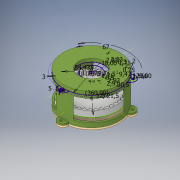
# Autodesk Inventor part: HarmonicDriveProto2
Saved by Autodesk Inventor 2018.3 (Build 223284000, 284)
## iProperties
Created: 2018-06-22
Part Number: HarmonicDriveProto2
Material: Generisch
Document SubType Name: Modeling
Designer: JochenAlt
Density: 1 g/cm^3
Appearance: Vorgabe
Author: JochenAlt
Autodesk Inventor part; units mm, degrees
note: some values were not read from the file. Chosen so that the rebuilt part matches the saved one: sketch regions of "Extrusion4".
(part 1 of 2)
sketch "Riemen" plane through (0, 0, 0) normal (0, 0, 1) x (1, 0, 0)
  circle A0 centre (0, 0) radius 26.0231 construction
  circle A1 centre (0, 0) radius 25.0331
  circle A2 centre (0, 0) radius 27.7331 construction
  line L0 (0, 43.2011) -> (0, -39.5773) construction
  line L1 (-38.8525, 0) -> (38.8525, 0) construction
  line L2 (0, 0) -> (5.5324, 31.3756) construction
  circle A3 centre (0, 0) radius 25.7831 construction
  line L3 (-1.465, 25.7414) -> (1.465, 25.7414) construction
  line L4 (3.0272, 25.6048) -> (5.9127, 25.096) construction
  arc A4 (4.0244, 27.3363) -> (3.1484, 26.0672) centre (5.9127, 25.096) ccw
  arc A5 (0.5595, 27.7275) -> (0, 27.7331) centre (0, 0) ccw
  arc A6 (4.8158, 27.3118) -> (4.2638, 27.4034) centre (0, 0) ccw
  arc A7 (2.8327, 25.8685) -> (1.7024, 25.9674) centre (0, 0) ccw
  arc A8 (1.426, 26.2179) -> (0.7837, 27.6198) centre (-1.465, 25.7414) ccw
  arc A9 (0.7837, 27.6198) -> (0.5595, 27.7275) centre (0.5534, 27.4275) ccw
  arc A10 (1.426, 26.2179) -> (1.7024, 25.9674) centre (1.722, 26.2667) ccw
  arc A11 (2.8327, 25.8685) -> (3.1484, 26.0672) centre (2.8653, 26.1667) ccw
  arc A12 (4.2638, 27.4034) -> (4.0244, 27.3363) centre (4.2177, 27.1069) ccw
  line L5 (0, 0) -> (2.7172, 31.0575) construction
  arc A13 (-4.2638, 27.4034) -> (-4.8158, 27.3118) centre (0, 0) ccw
  arc A14 (-4.0244, 27.3363) -> (-4.2638, 27.4034) centre (-4.2177, 27.1069) ccw
  arc A15 (-3.1484, 26.0672) -> (-4.0244, 27.3363) centre (-5.9127, 25.096) ccw
  arc A16 (-3.1484, 26.0672) -> (-2.8327, 25.8685) centre (-2.8653, 26.1667) ccw
  arc A17 (-1.7024, 25.9674) -> (-2.8327, 25.8685) centre (0, 0) ccw
  arc A18 (-1.7024, 25.9674) -> (-1.426, 26.2179) centre (-1.722, 26.2667) ccw
  arc A19 (-0.7837, 27.6198) -> (-1.426, 26.2179) centre (1.465, 25.7414) ccw
  arc A20 (-0.5595, 27.7275) -> (-0.7837, 27.6198) centre (-0.5534, 27.4275) ccw
  arc A21 (0, 27.7331) -> (-0.5595, 27.7275) centre (0, 0) ccw
  arc A22 (-8.9576, 26.2466) -> (-9.4853, 26.0606) centre (0, 0) ccw
  arc A23 (-8.7101, 26.2222) -> (-8.9576, 26.2466) centre (-8.8607, 25.9627) ccw
  arc A24 (-7.6271, 25.1245) -> (-8.7101, 26.2222) centre (-10.1807, 23.688) ccw
  arc A25 (-7.6271, 25.1245) -> (-7.2816, 24.9836) centre (-7.3656, 25.2716) ccw
  arc A26 (-6.1857, 25.2772) -> (-7.2816, 24.9836) centre (0, 0) ccw
  arc A27 (-6.1857, 25.2772) -> (-5.957, 25.572) centre (-6.257, 25.5686) ccw
  arc A28 (-5.5679, 27.0642) -> (-5.957, 25.572) centre (-3.0272, 25.6048) ccw
  arc A29 (-5.3658, 27.2091) -> (-5.5679, 27.0642) centre (-5.3078, 26.9147) ccw
  arc A30 (-4.8158, 27.3118) -> (-5.3658, 27.2091) centre (0, 0) ccw
  arc A31 (-13.3792, 24.2924) -> (-13.8666, 24.0176) centre (0, 0) ccw
  arc A32 (-13.1312, 24.3113) -> (-13.3792, 24.2924) centre (-13.2345, 24.0296) ccw
  arc A33 (-11.874, 23.4184) -> (-13.1312, 24.3113) centre (-14.1395, 21.5602) ccw
  arc A34 (-11.874, 23.4184) -> (-11.5094, 23.3396) centre (-11.6421, 23.6086) ccw
  arc A35 (-10.4811, 23.8191) -> (-11.5094, 23.3396) centre (0, 0) ccw
  arc A36 (-10.4811, 23.8191) -> (-10.3071, 24.1491) centre (-10.6019, 24.0937) ccw
  arc A37 (-10.183, 25.6861) -> (-10.3071, 24.1491) centre (-7.4274, 24.6901) ccw
  arc A38 (-10.0091, 25.8639) -> (-10.183, 25.6861) centre (-9.9008, 25.5842) ccw
  arc A39 (-9.4853, 26.0606) -> (-10.0091, 25.8639) centre (0, 0) ccw
  arc A40 (-17.3943, 21.6001) -> (-17.8265, 21.2448) centre (0, 0) ccw
  arc A41 (-17.1534, 21.6618) -> (-17.3943, 21.6001) centre (-17.2061, 21.3664) ccw
  arc A42 (-15.7602, 21.0007) -> (-17.1534, 21.6618) centre (-17.6685, 18.7774) ccw
  arc A43 (-15.7602, 21.0007) -> (-15.3874, 20.9864) centre (-15.5648, 21.2284) ccw
  arc A44 (-14.458, 21.6372) -> (-15.3874, 20.9864) centre (0, 0) ccw
  arc A45 (-14.458, 21.6372) -> (-14.3439, 21.9924) centre (-14.6247, 21.8866) ccw
  arc A46 (-14.4886, 23.5277) -> (-14.3439, 21.9924) centre (-11.602, 23.0252) ccw
  arc A47 (-14.3483, 23.7329) -> (-14.4886, 23.5277) centre (-14.193, 23.4762) ccw
  arc A48 (-13.8666, 24.0176) -> (-14.3483, 23.7329) centre (0, 0) ccw
  arc A49 (-20.8808, 18.2515) -> (-21.2448, 17.8265) centre (0, 0) ccw
  arc A50 (-20.6543, 18.354) -> (-20.8808, 18.2515) centre (-20.655, 18.054) ccw
  arc A51 (-19.1675, 17.9449) -> (-20.6543, 18.354) centre (-20.6608, 15.424) ccw
  arc A52 (-19.1675, 17.9449) -> (-18.7979, 17.9956) centre (-19.0146, 18.2031) ccw
  arc A53 (-17.9956, 18.7979) -> (-18.7979, 17.9956) centre (0, 0) ccw
  arc A54 (-17.9956, 18.7979) -> (-17.9449, 19.1675) centre (-18.2031, 19.0146) ccw
  arc A55 (-18.354, 20.6543) -> (-17.9449, 19.1675) centre (-15.424, 20.6608) ccw
  arc A56 (-18.2515, 20.8808) -> (-18.354, 20.6543) centre (-18.054, 20.655) ccw
  arc A57 (-17.8265, 21.2448) -> (-18.2515, 20.8808) centre (0, 0) ccw
  arc A58 (-23.7329, 14.3483) -> (-24.0176, 13.8666) centre (0, 0) ccw
  arc A59 (-23.5277, 14.4886) -> (-23.7329, 14.3483) centre (-23.4762, 14.193) ccw
  arc A60 (-21.9924, 14.3439) -> (-23.5277, 14.4886) centre (-23.0252, 11.602) ccw
  arc A61 (-21.9924, 14.3439) -> (-21.6372, 14.458) centre (-21.8866, 14.6247) ccw
  arc A62 (-20.9864, 15.3874) -> (-21.6372, 14.458) centre (0, 0) ccw
  arc A63 (-20.9864, 15.3874) -> (-21.0007, 15.7602) centre (-21.2284, 15.5648) ccw
  arc A64 (-21.6618, 17.1534) -> (-21.0007, 15.7602) centre (-18.7774, 17.6685) ccw
  arc A65 (-21.6001, 17.3943) -> (-21.6618, 17.1534) centre (-21.3664, 17.2061) ccw
  arc A66 (-21.2448, 17.8265) -> (-21.6001, 17.3943) centre (0, 0) ccw
  arc A67 (-25.8639, 10.0091) -> (-26.0606, 9.4853) centre (0, 0) ccw
  arc A68 (-25.6861, 10.183) -> (-25.8639, 10.0091) centre (-25.5842, 9.9008) ccw
  arc A69 (-24.1491, 10.3071) -> (-25.6861, 10.183) centre (-24.6901, 7.4274) ccw
  arc A70 (-24.1491, 10.3071) -> (-23.8191, 10.4811) centre (-24.0937, 10.6019) ccw
  arc A71 (-23.3396, 11.5094) -> (-23.8191, 10.4811) centre (0, 0) ccw
  arc A72 (-23.3396, 11.5094) -> (-23.4184, 11.874) centre (-23.6086, 11.6421) ccw
  arc A73 (-24.3113, 13.1312) -> (-23.4184, 11.874) centre (-21.5602, 14.1395) ccw
  arc A74 (-24.2924, 13.3792) -> (-24.3113, 13.1312) centre (-24.0296, 13.2345) ccw
  arc A75 (-24.0176, 13.8666) -> (-24.2924, 13.3792) centre (0, 0) ccw
  arc A76 (-27.2091, 5.3658) -> (-27.3118, 4.8158) centre (0, 0) ccw
  arc A77 (-27.0642, 5.5679) -> (-27.2091, 5.3658) centre (-26.9147, 5.3078) ccw
  arc A78 (-25.572, 5.957) -> (-27.0642, 5.5679) centre (-25.6048, 3.0272) ccw
  arc A79 (-25.572, 5.957) -> (-25.2772, 6.1857) centre (-25.5686, 6.257) ccw
  arc A80 (-24.9836, 7.2816) -> (-25.2772, 6.1857) centre (0, 0) ccw
  arc A81 (-24.9836, 7.2816) -> (-25.1245, 7.6271) centre (-25.2716, 7.3656) ccw
  arc A82 (-26.2222, 8.7101) -> (-25.1245, 7.6271) centre (-23.688, 10.1807) ccw
  arc A83 (-26.2466, 8.9576) -> (-26.2222, 8.7101) centre (-25.9627, 8.8607) ccw
  arc A84 (-26.0606, 9.4853) -> (-26.2466, 8.9576) centre (0, 0) ccw
  arc A85 (-27.7275, 0.5595) -> (-27.7331, 0) centre (0, 0) ccw
  arc A86 (-27.6198, 0.7837) -> (-27.7275, 0.5595) centre (-27.4275, 0.5534) ccw
  arc A87 (-26.2179, 1.426) -> (-27.6198, 0.7837) centre (-25.7414, -1.465) ccw
  arc A88 (-26.2179, 1.426) -> (-25.9674, 1.7024) centre (-26.2667, 1.722) ccw
  arc A89 (-25.8685, 2.8327) -> (-25.9674, 1.7024) centre (0, 0) ccw
  arc A90 (-25.8685, 2.8327) -> (-26.0672, 3.1484) centre (-26.1667, 2.8653) ccw
  arc A91 (-27.3363, 4.0244) -> (-26.0672, 3.1484) centre (-25.096, 5.9127) ccw
  arc A92 (-27.4034, 4.2638) -> (-27.3363, 4.0244) centre (-27.1069, 4.2177) ccw
  arc A93 (-27.3118, 4.8158) -> (-27.4034, 4.2638) centre (0, 0) ccw
  arc A94 (-27.4034, -4.2638) -> (-27.3118, -4.8158) centre (0, 0) ccw
  arc A95 (-27.3363, -4.0244) -> (-27.4034, -4.2638) centre (-27.1069, -4.2177) ccw
  arc A96 (-26.0672, -3.1484) -> (-27.3363, -4.0244) centre (-25.096, -5.9127) ccw
  arc A97 (-26.0672, -3.1484) -> (-25.8685, -2.8327) centre (-26.1667, -2.8653) ccw
  arc A98 (-25.9674, -1.7024) -> (-25.8685, -2.8327) centre (0, 0) ccw
  arc A99 (-25.9674, -1.7024) -> (-26.2179, -1.426) centre (-26.2667, -1.722) ccw
  arc A100 (-27.6198, -0.7837) -> (-26.2179, -1.426) centre (-25.7414, 1.465) ccw
  arc A101 (-27.7275, -0.5595) -> (-27.6198, -0.7837) centre (-27.4275, -0.5534) ccw
  arc A102 (-27.7331, 0) -> (-27.7275, -0.5595) centre (0, 0) ccw
  arc A103 (-26.2466, -8.9576) -> (-26.0606, -9.4853) centre (0, 0) ccw
  arc A104 (-26.2222, -8.7101) -> (-26.2466, -8.9576) centre (-25.9627, -8.8607) ccw
  arc A105 (-25.1245, -7.6271) -> (-26.2222, -8.7101) centre (-23.688, -10.1807) ccw
  arc A106 (-25.1245, -7.6271) -> (-24.9836, -7.2816) centre (-25.2716, -7.3656) ccw
  arc A107 (-25.2772, -6.1857) -> (-24.9836, -7.2816) centre (0, 0) ccw
  arc A108 (-25.2772, -6.1857) -> (-25.572, -5.957) centre (-25.5686, -6.257) ccw
  arc A109 (-27.0642, -5.5679) -> (-25.572, -5.957) centre (-25.6048, -3.0272) ccw
  arc A110 (-27.2091, -5.3658) -> (-27.0642, -5.5679) centre (-26.9147, -5.3078) ccw
  arc A111 (-27.3118, -4.8158) -> (-27.2091, -5.3658) centre (0, 0) ccw
  arc A112 (-24.2924, -13.3792) -> (-24.0176, -13.8666) centre (0, 0) ccw
  arc A113 (-24.3113, -13.1312) -> (-24.2924, -13.3792) centre (-24.0296, -13.2345) ccw
  arc A114 (-23.4184, -11.874) -> (-24.3113, -13.1312) centre (-21.5602, -14.1395) ccw
  arc A115 (-23.4184, -11.874) -> (-23.3396, -11.5094) centre (-23.6086, -11.6421) ccw
  arc A116 (-23.8191, -10.4811) -> (-23.3396, -11.5094) centre (0, 0) ccw
  arc A117 (-23.8191, -10.4811) -> (-24.1491, -10.3071) centre (-24.0937, -10.6019) ccw
  arc A118 (-25.6861, -10.183) -> (-24.1491, -10.3071) centre (-24.6901, -7.4274) ccw
  arc A119 (-25.8639, -10.0091) -> (-25.6861, -10.183) centre (-25.5842, -9.9008) ccw
  arc A120 (-26.0606, -9.4853) -> (-25.8639, -10.0091) centre (0, 0) ccw
  arc A121 (-21.6001, -17.3943) -> (-21.2448, -17.8265) centre (0, 0) ccw
  arc A122 (-21.6618, -17.1534) -> (-21.6001, -17.3943) centre (-21.3664, -17.2061) ccw
  arc A123 (-21.0007, -15.7602) -> (-21.6618, -17.1534) centre (-18.7774, -17.6685) ccw
  arc A124 (-21.0007, -15.7602) -> (-20.9864, -15.3874) centre (-21.2284, -15.5648) ccw
  arc A125 (-21.6372, -14.458) -> (-20.9864, -15.3874) centre (0, 0) ccw
  arc A126 (-21.6372, -14.458) -> (-21.9924, -14.3439) centre (-21.8866, -14.6247) ccw
  arc A127 (-23.5277, -14.4886) -> (-21.9924, -14.3439) centre (-23.0252, -11.602) ccw
  arc A128 (-23.7329, -14.3483) -> (-23.5277, -14.4886) centre (-23.4762, -14.193) ccw
  arc A129 (-24.0176, -13.8666) -> (-23.7329, -14.3483) centre (0, 0) ccw
  arc A130 (-18.2515, -20.8808) -> (-17.8265, -21.2448) centre (0, 0) ccw
  arc A131 (-18.354, -20.6543) -> (-18.2515, -20.8808) centre (-18.054, -20.655) ccw
  arc A132 (-17.9449, -19.1675) -> (-18.354, -20.6543) centre (-15.424, -20.6608) ccw
  arc A133 (-17.9449, -19.1675) -> (-17.9956, -18.7979) centre (-18.2031, -19.0146) ccw
  arc A134 (-18.7979, -17.9956) -> (-17.9956, -18.7979) centre (0, 0) ccw
  arc A135 (-18.7979, -17.9956) -> (-19.1675, -17.9449) centre (-19.0146, -18.2031) ccw
  arc A136 (-20.6543, -18.354) -> (-19.1675, -17.9449) centre (-20.6608, -15.424) ccw
  arc A137 (-20.8808, -18.2515) -> (-20.6543, -18.354) centre (-20.655, -18.054) ccw
  arc A138 (-21.2448, -17.8265) -> (-20.8808, -18.2515) centre (0, 0) ccw
  arc A139 (-14.3483, -23.7329) -> (-13.8666, -24.0176) centre (0, 0) ccw
  arc A140 (-14.4886, -23.5277) -> (-14.3483, -23.7329) centre (-14.193, -23.4762) ccw
  arc A141 (-14.3439, -21.9924) -> (-14.4886, -23.5277) centre (-11.602, -23.0252) ccw
  arc A142 (-14.3439, -21.9924) -> (-14.458, -21.6372) centre (-14.6247, -21.8866) ccw
  arc A143 (-15.3874, -20.9864) -> (-14.458, -21.6372) centre (0, 0) ccw
  arc A144 (-15.3874, -20.9864) -> (-15.7602, -21.0007) centre (-15.5648, -21.2284) ccw
  arc A145 (-17.1534, -21.6618) -> (-15.7602, -21.0007) centre (-17.6685, -18.7774) ccw
  arc A146 (-17.3943, -21.6001) -> (-17.1534, -21.6618) centre (-17.2061, -21.3664) ccw
  arc A147 (-17.8265, -21.2448) -> (-17.3943, -21.6001) centre (0, 0) ccw
  arc A148 (-10.0091, -25.8639) -> (-9.4853, -26.0606) centre (0, 0) ccw
  arc A149 (-10.183, -25.6861) -> (-10.0091, -25.8639) centre (-9.9008, -25.5842) ccw
  arc A150 (-10.3071, -24.1491) -> (-10.183, -25.6861) centre (-7.4274, -24.6901) ccw
  arc A151 (-10.3071, -24.1491) -> (-10.4811, -23.8191) centre (-10.6019, -24.0937) ccw
  arc A152 (-11.5094, -23.3396) -> (-10.4811, -23.8191) centre (0, 0) ccw
  arc A153 (-11.5094, -23.3396) -> (-11.874, -23.4184) centre (-11.6421, -23.6086) ccw
  arc A154 (-13.1312, -24.3113) -> (-11.874, -23.4184) centre (-14.1395, -21.5602) ccw
  arc A155 (-13.3792, -24.2924) -> (-13.1312, -24.3113) centre (-13.2345, -24.0296) ccw
  arc A156 (-13.8666, -24.0176) -> (-13.3792, -24.2924) centre (0, 0) ccw
  arc A157 (-5.3658, -27.2091) -> (-4.8158, -27.3118) centre (0, 0) ccw
  arc A158 (-5.5679, -27.0642) -> (-5.3658, -27.2091) centre (-5.3078, -26.9147) ccw
  arc A159 (-5.957, -25.572) -> (-5.5679, -27.0642) centre (-3.0272, -25.6048) ccw
  arc A160 (-5.957, -25.572) -> (-6.1857, -25.2772) centre (-6.257, -25.5686) ccw
  arc A161 (-7.2816, -24.9836) -> (-6.1857, -25.2772) centre (0, 0) ccw
  arc A162 (-7.2816, -24.9836) -> (-7.6271, -25.1245) centre (-7.3656, -25.2716) ccw
  arc A163 (-8.7101, -26.2222) -> (-7.6271, -25.1245) centre (-10.1807, -23.688) ccw
  arc A164 (-8.9576, -26.2466) -> (-8.7101, -26.2222) centre (-8.8607, -25.9627) ccw
  arc A165 (-9.4853, -26.0606) -> (-8.9576, -26.2466) centre (0, 0) ccw
  arc A166 (-0.5595, -27.7275) -> (0, -27.7331) centre (0, 0) ccw
  arc A167 (-0.7837, -27.6198) -> (-0.5595, -27.7275) centre (-0.5534, -27.4275) ccw
  arc A168 (-1.426, -26.2179) -> (-0.7837, -27.6198) centre (1.465, -25.7414) ccw
  arc A169 (-1.426, -26.2179) -> (-1.7024, -25.9674) centre (-1.722, -26.2667) ccw
  arc A170 (-2.8327, -25.8685) -> (-1.7024, -25.9674) centre (0, 0) ccw
  arc A171 (-2.8327, -25.8685) -> (-3.1484, -26.0672) centre (-2.8653, -26.1667) ccw
  arc A172 (-4.0244, -27.3363) -> (-3.1484, -26.0672) centre (-5.9127, -25.096) ccw
  arc A173 (-4.2638, -27.4034) -> (-4.0244, -27.3363) centre (-4.2177, -27.1069) ccw
  arc A174 (-4.8158, -27.3118) -> (-4.2638, -27.4034) centre (0, 0) ccw
  arc A175 (4.2638, -27.4034) -> (4.8158, -27.3118) centre (0, 0) ccw
  arc A176 (4.0244, -27.3363) -> (4.2638, -27.4034) centre (4.2177, -27.1069) ccw
  arc A177 (3.1484, -26.0672) -> (4.0244, -27.3363) centre (5.9127, -25.096) ccw
  arc A178 (3.1484, -26.0672) -> (2.8327, -25.8685) centre (2.8653, -26.1667) ccw
  arc A179 (1.7024, -25.9674) -> (2.8327, -25.8685) centre (0, 0) ccw
  arc A180 (1.7024, -25.9674) -> (1.426, -26.2179) centre (1.722, -26.2667) ccw
  arc A181 (0.7837, -27.6198) -> (1.426, -26.2179) centre (-1.465, -25.7414) ccw
  arc A182 (0.5595, -27.7275) -> (0.7837, -27.6198) centre (0.5534, -27.4275) ccw
  arc A183 (0, -27.7331) -> (0.5595, -27.7275) centre (0, 0) ccw
  arc A184 (8.9576, -26.2466) -> (9.4853, -26.0606) centre (0, 0) ccw
  arc A185 (8.7101, -26.2222) -> (8.9576, -26.2466) centre (8.8607, -25.9627) ccw
  arc A186 (7.6271, -25.1245) -> (8.7101, -26.2222) centre (10.1807, -23.688) ccw
  arc A187 (7.6271, -25.1245) -> (7.2816, -24.9836) centre (7.3656, -25.2716) ccw
  arc A188 (6.1857, -25.2772) -> (7.2816, -24.9836) centre (0, 0) ccw
  arc A189 (6.1857, -25.2772) -> (5.957, -25.572) centre (6.257, -25.5686) ccw
  arc A190 (5.5679, -27.0642) -> (5.957, -25.572) centre (3.0272, -25.6048) ccw
  arc A191 (5.3658, -27.2091) -> (5.5679, -27.0642) centre (5.3078, -26.9147) ccw
  arc A192 (4.8158, -27.3118) -> (5.3658, -27.2091) centre (0, 0) ccw
  arc A193 (13.3792, -24.2924) -> (13.8666, -24.0176) centre (0, 0) ccw
  arc A194 (13.1312, -24.3113) -> (13.3792, -24.2924) centre (13.2345, -24.0296) ccw
  arc A195 (11.874, -23.4184) -> (13.1312, -24.3113) centre (14.1395, -21.5602) ccw
  arc A196 (11.874, -23.4184) -> (11.5094, -23.3396) centre (11.6421, -23.6086) ccw
  arc A197 (10.4811, -23.8191) -> (11.5094, -23.3396) centre (0, 0) ccw
  arc A198 (10.4811, -23.8191) -> (10.3071, -24.1491) centre (10.6019, -24.0937) ccw
  arc A199 (10.183, -25.6861) -> (10.3071, -24.1491) centre (7.4274, -24.6901) ccw
  arc A200 (10.0091, -25.8639) -> (10.183, -25.6861) centre (9.9008, -25.5842) ccw
  arc A201 (9.4853, -26.0606) -> (10.0091, -25.8639) centre (0, 0) ccw
  arc A202 (17.3943, -21.6001) -> (17.8265, -21.2448) centre (0, 0) ccw
  arc A203 (17.1534, -21.6618) -> (17.3943, -21.6001) centre (17.2061, -21.3664) ccw
  arc A204 (15.7602, -21.0007) -> (17.1534, -21.6618) centre (17.6685, -18.7774) ccw
  arc A205 (15.7602, -21.0007) -> (15.3874, -20.9864) centre (15.5648, -21.2284) ccw
  arc A206 (14.458, -21.6372) -> (15.3874, -20.9864) centre (0, 0) ccw
  arc A207 (14.458, -21.6372) -> (14.3439, -21.9924) centre (14.6247, -21.8866) ccw
  arc A208 (14.4886, -23.5277) -> (14.3439, -21.9924) centre (11.602, -23.0252) ccw
  arc A209 (14.3483, -23.7329) -> (14.4886, -23.5277) centre (14.193, -23.4762) ccw
  arc A210 (13.8666, -24.0176) -> (14.3483, -23.7329) centre (0, 0) ccw
  arc A211 (20.8808, -18.2515) -> (21.2448, -17.8265) centre (0, 0) ccw
  arc A212 (20.6543, -18.354) -> (20.8808, -18.2515) centre (20.655, -18.054) ccw
  arc A213 (19.1675, -17.9449) -> (20.6543, -18.354) centre (20.6608, -15.424) ccw
  arc A214 (19.1675, -17.9449) -> (18.7979, -17.9956) centre (19.0146, -18.2031) ccw
  arc A215 (17.9956, -18.7979) -> (18.7979, -17.9956) centre (0, 0) ccw
  arc A216 (17.9956, -18.7979) -> (17.9449, -19.1675) centre (18.2031, -19.0146) ccw
  arc A217 (18.354, -20.6543) -> (17.9449, -19.1675) centre (15.424, -20.6608) ccw
  arc A218 (18.2515, -20.8808) -> (18.354, -20.6543) centre (18.054, -20.655) ccw
  arc A219 (17.8265, -21.2448) -> (18.2515, -20.8808) centre (0, 0) ccw
  arc A220 (23.7329, -14.3483) -> (24.0176, -13.8666) centre (0, 0) ccw
  arc A221 (23.5277, -14.4886) -> (23.7329, -14.3483) centre (23.4762, -14.193) ccw
  arc A222 (21.9924, -14.3439) -> (23.5277, -14.4886) centre (23.0252, -11.602) ccw
  arc A223 (21.9924, -14.3439) -> (21.6372, -14.458) centre (21.8866, -14.6247) ccw
  arc A224 (20.9864, -15.3874) -> (21.6372, -14.458) centre (0, 0) ccw
  arc A225 (20.9864, -15.3874) -> (21.0007, -15.7602) centre (21.2284, -15.5648) ccw
  arc A226 (21.6618, -17.1534) -> (21.0007, -15.7602) centre (18.7774, -17.6685) ccw
  arc A227 (21.6001, -17.3943) -> (21.6618, -17.1534) centre (21.3664, -17.2061) ccw
  arc A228 (21.2448, -17.8265) -> (21.6001, -17.3943) centre (0, 0) ccw
  arc A229 (25.8639, -10.0091) -> (26.0606, -9.4853) centre (0, 0) ccw
  arc A230 (25.6861, -10.183) -> (25.8639, -10.0091) centre (25.5842, -9.9008) ccw
  arc A231 (24.1491, -10.3071) -> (25.6861, -10.183) centre (24.6901, -7.4274) ccw
  arc A232 (24.1491, -10.3071) -> (23.8191, -10.4811) centre (24.0937, -10.6019) ccw
  arc A233 (23.3396, -11.5094) -> (23.8191, -10.4811) centre (0, 0) ccw
  arc A234 (23.3396, -11.5094) -> (23.4184, -11.874) centre (23.6086, -11.6421) ccw
  arc A235 (24.3113, -13.1312) -> (23.4184, -11.874) centre (21.5602, -14.1395) ccw
  arc A236 (24.2924, -13.3792) -> (24.3113, -13.1312) centre (24.0296, -13.2345) ccw
  arc A237 (24.0176, -13.8666) -> (24.2924, -13.3792) centre (0, 0) ccw
  arc A238 (27.2091, -5.3658) -> (27.3118, -4.8158) centre (0, 0) ccw
  arc A239 (27.0642, -5.5679) -> (27.2091, -5.3658) centre (26.9147, -5.3078) ccw
  arc A240 (25.572, -5.957) -> (27.0642, -5.5679) centre (25.6048, -3.0272) ccw
  arc A241 (25.572, -5.957) -> (25.2772, -6.1857) centre (25.5686, -6.257) ccw
  arc A242 (24.9836, -7.2816) -> (25.2772, -6.1857) centre (0, 0) ccw
  arc A243 (24.9836, -7.2816) -> (25.1245, -7.6271) centre (25.2716, -7.3656) ccw
  arc A244 (26.2222, -8.7101) -> (25.1245, -7.6271) centre (23.688, -10.1807) ccw
  arc A245 (26.2466, -8.9576) -> (26.2222, -8.7101) centre (25.9627, -8.8607) ccw
  arc A246 (26.0606, -9.4853) -> (26.2466, -8.9576) centre (0, 0) ccw
  arc A247 (27.7275, -0.5595) -> (27.7331, 0) centre (0, 0) ccw
  arc A248 (27.6198, -0.7837) -> (27.7275, -0.5595) centre (27.4275, -0.5534) ccw
  arc A249 (26.2179, -1.426) -> (27.6198, -0.7837) centre (25.7414, 1.465) ccw
  arc A250 (26.2179, -1.426) -> (25.9674, -1.7024) centre (26.2667, -1.722) ccw
  arc A251 (25.8685, -2.8327) -> (25.9674, -1.7024) centre (0, 0) ccw
  arc A252 (25.8685, -2.8327) -> (26.0672, -3.1484) centre (26.1667, -2.8653) ccw
  arc A253 (27.3363, -4.0244) -> (26.0672, -3.1484) centre (25.096, -5.9127) ccw
  arc A254 (27.4034, -4.2638) -> (27.3363, -4.0244) centre (27.1069, -4.2177) ccw
  arc A255 (27.3118, -4.8158) -> (27.4034, -4.2638) centre (0, 0) ccw
  arc A256 (27.4034, 4.2638) -> (27.3118, 4.8158) centre (0, 0) ccw
  arc A257 (27.3363, 4.0244) -> (27.4034, 4.2638) centre (27.1069, 4.2177) ccw
  arc A258 (26.0672, 3.1484) -> (27.3363, 4.0244) centre (25.096, 5.9127) ccw
  arc A259 (26.0672, 3.1484) -> (25.8685, 2.8327) centre (26.1667, 2.8653) ccw
  arc A260 (25.9674, 1.7024) -> (25.8685, 2.8327) centre (0, 0) ccw
  arc A261 (25.9674, 1.7024) -> (26.2179, 1.426) centre (26.2667, 1.722) ccw
  arc A262 (27.6198, 0.7837) -> (26.2179, 1.426) centre (25.7414, -1.465) ccw
  arc A263 (27.7275, 0.5595) -> (27.6198, 0.7837) centre (27.4275, 0.5534) ccw
  arc A264 (27.7331, 0) -> (27.7275, 0.5595) centre (0, 0) ccw
  arc A265 (26.2466, 8.9576) -> (26.0606, 9.4853) centre (0, 0) ccw
  arc A266 (26.2222, 8.7101) -> (26.2466, 8.9576) centre (25.9627, 8.8607) ccw
  arc A267 (25.1245, 7.6271) -> (26.2222, 8.7101) centre (23.688, 10.1807) ccw
  arc A268 (25.1245, 7.6271) -> (24.9836, 7.2816) centre (25.2716, 7.3656) ccw
  arc A269 (25.2772, 6.1857) -> (24.9836, 7.2816) centre (0, 0) ccw
  arc A270 (25.2772, 6.1857) -> (25.572, 5.957) centre (25.5686, 6.257) ccw
  arc A271 (27.0642, 5.5679) -> (25.572, 5.957) centre (25.6048, 3.0272) ccw
  arc A272 (27.2091, 5.3658) -> (27.0642, 5.5679) centre (26.9147, 5.3078) ccw
  arc A273 (27.3118, 4.8158) -> (27.2091, 5.3658) centre (0, 0) ccw
  arc A274 (24.2924, 13.3792) -> (24.0176, 13.8666) centre (0, 0) ccw
  arc A275 (24.3113, 13.1312) -> (24.2924, 13.3792) centre (24.0296, 13.2345) ccw
  arc A276 (23.4184, 11.874) -> (24.3113, 13.1312) centre (21.5602, 14.1395) ccw
  arc A277 (23.4184, 11.874) -> (23.3396, 11.5094) centre (23.6086, 11.6421) ccw
  arc A278 (23.8191, 10.4811) -> (23.3396, 11.5094) centre (0, 0) ccw
  arc A279 (23.8191, 10.4811) -> (24.1491, 10.3071) centre (24.0937, 10.6019) ccw
  arc A280 (25.6861, 10.183) -> (24.1491, 10.3071) centre (24.6901, 7.4274) ccw
  arc A281 (25.8639, 10.0091) -> (25.6861, 10.183) centre (25.5842, 9.9008) ccw
  arc A282 (26.0606, 9.4853) -> (25.8639, 10.0091) centre (0, 0) ccw
  arc A283 (21.6001, 17.3943) -> (21.2448, 17.8265) centre (0, 0) ccw
  arc A284 (21.6618, 17.1534) -> (21.6001, 17.3943) centre (21.3664, 17.2061) ccw
  arc A285 (21.0007, 15.7602) -> (21.6618, 17.1534) centre (18.7774, 17.6685) ccw
  arc A286 (21.0007, 15.7602) -> (20.9864, 15.3874) centre (21.2284, 15.5648) ccw
  arc A287 (21.6372, 14.458) -> (20.9864, 15.3874) centre (0, 0) ccw
  arc A288 (21.6372, 14.458) -> (21.9924, 14.3439) centre (21.8866, 14.6247) ccw
  arc A289 (23.5277, 14.4886) -> (21.9924, 14.3439) centre (23.0252, 11.602) ccw
  arc A290 (23.7329, 14.3483) -> (23.5277, 14.4886) centre (23.4762, 14.193) ccw
  arc A291 (24.0176, 13.8666) -> (23.7329, 14.3483) centre (0, 0) ccw
  arc A292 (18.2515, 20.8808) -> (17.8265, 21.2448) centre (0, 0) ccw
  arc A293 (18.354, 20.6543) -> (18.2515, 20.8808) centre (18.054, 20.655) ccw
  arc A294 (17.9449, 19.1675) -> (18.354, 20.6543) centre (15.424, 20.6608) ccw
  arc A295 (17.9449, 19.1675) -> (17.9956, 18.7979) centre (18.2031, 19.0146) ccw
  arc A296 (18.7979, 17.9956) -> (17.9956, 18.7979) centre (0, 0) ccw
  arc A297 (18.7979, 17.9956) -> (19.1675, 17.9449) centre (19.0146, 18.2031) ccw
  arc A298 (20.6543, 18.354) -> (19.1675, 17.9449) centre (20.6608, 15.424) ccw
  arc A299 (20.8808, 18.2515) -> (20.6543, 18.354) centre (20.655, 18.054) ccw
  arc A300 (21.2448, 17.8265) -> (20.8808, 18.2515) centre (0, 0) ccw
  arc A301 (14.3483, 23.7329) -> (13.8666, 24.0176) centre (0, 0) ccw
  arc A302 (14.4886, 23.5277) -> (14.3483, 23.7329) centre (14.193, 23.4762) ccw
  arc A303 (14.3439, 21.9924) -> (14.4886, 23.5277) centre (11.602, 23.0252) ccw
  arc A304 (14.3439, 21.9924) -> (14.458, 21.6372) centre (14.6247, 21.8866) ccw
  arc A305 (15.3874, 20.9864) -> (14.458, 21.6372) centre (0, 0) ccw
  arc A306 (15.3874, 20.9864) -> (15.7602, 21.0007) centre (15.5648, 21.2284) ccw
  arc A307 (17.1534, 21.6618) -> (15.7602, 21.0007) centre (17.6685, 18.7774) ccw
  arc A308 (17.3943, 21.6001) -> (17.1534, 21.6618) centre (17.2061, 21.3664) ccw
  arc A309 (17.8265, 21.2448) -> (17.3943, 21.6001) centre (0, 0) ccw
  arc A310 (10.0091, 25.8639) -> (9.4853, 26.0606) centre (0, 0) ccw
  arc A311 (10.183, 25.6861) -> (10.0091, 25.8639) centre (9.9008, 25.5842) ccw
  arc A312 (10.3071, 24.1491) -> (10.183, 25.6861) centre (7.4274, 24.6901) ccw
  arc A313 (10.3071, 24.1491) -> (10.4811, 23.8191) centre (10.6019, 24.0937) ccw
  arc A314 (11.5094, 23.3396) -> (10.4811, 23.8191) centre (0, 0) ccw
  arc A315 (11.5094, 23.3396) -> (11.874, 23.4184) centre (11.6421, 23.6086) ccw
  arc A316 (13.1312, 24.3113) -> (11.874, 23.4184) centre (14.1395, 21.5602) ccw
  arc A317 (13.3792, 24.2924) -> (13.1312, 24.3113) centre (13.2345, 24.0296) ccw
  arc A318 (13.8666, 24.0176) -> (13.3792, 24.2924) centre (0, 0) ccw
  arc A319 (5.3658, 27.2091) -> (4.8158, 27.3118) centre (0, 0) ccw
  arc A320 (5.5679, 27.0642) -> (5.3658, 27.2091) centre (5.3078, 26.9147) ccw
  arc A321 (5.957, 25.572) -> (5.5679, 27.0642) centre (3.0272, 25.6048) ccw
  arc A322 (5.957, 25.572) -> (6.1857, 25.2772) centre (6.257, 25.5686) ccw
  arc A323 (7.2816, 24.9836) -> (6.1857, 25.2772) centre (0, 0) ccw
  arc A324 (7.2816, 24.9836) -> (7.6271, 25.1245) centre (7.3656, 25.2716) ccw
  arc A325 (8.7101, 26.2222) -> (7.6271, 25.1245) centre (10.1807, 23.688) ccw
  arc A326 (8.9576, 26.2466) -> (8.7101, 26.2222) centre (8.8607, 25.9627) ccw
  arc A327 (9.4853, 26.0606) -> (8.9576, 26.2466) centre (0, 0) ccw
  point P0 (0, 26.0231)
  point P1 (4.5189, 25.6278)
  dimension "d0" = 10
  dimension "d258" = 1.71
  dimension "d259" = 2.7
  dimension "d260" = 0.75
  dimension "d261" = 51.5662
  dimension "d262" = 2.93
  dimension "d264" = 0.3
  dimension "d265" = 2.93
  constraints: 660 point on circle, 328 centre point, 8 end point, 8 tangent, 6 coincident, 6 equal radius, 4 point on line, 1 equal length, 1 horizontal, 1 symmetric about line, 2 other
  measures "d0" angle of L2 L0
  measures "d258" radial gap between concentric circles of A2 A0
  measures "d259" radial gap between concentric circles of A2 A1
  measures "d260" radial gap between concentric circles of A3 A1
  measures "d261" diameter of A3
  measures "d262" distance of L3.start L3.end
  measures "d264" radius of A9
  measures "d265" radius of A8
sketch "Enclosure" plane through (0, 0, 0) normal (0, 0, 1) x (1, 0, 0)
  circle A0 centre (0, 0) radius 2
  circle A1 centre (0, 0) radius 33.5
  circle A2 centre (0, 0) radius 15.25
  circle A3 centre (0, 0) radius 31.5
  line L0 (0, 51.8) -> (0, -55.3) construction
  circle A4 centre (0, -36.5) radius 1.5
  circle A5 centre (-31.6099, 18.25) radius 1.5
  circle A6 centre (31.6099, 18.25) radius 1.5
  circle A7 centre (0, 0) radius 36.5 construction
  line L1 (5.5282, -31.0111) -> (5.8792, -32.9801) construction
  line L2 (-5.5282, -31.0111) -> (-5.8792, -32.9801) construction
  circle A8 centre (31.6099, 18.25) radius 2.5
  circle A9 centre (-31.6099, 18.25) radius 2.5
  circle A10 centre (0, -36.5) radius 2.5
  line L3 (0, 0) -> (-31.6099, 18.25) construction
  line L4 (31.6099, 18.25) -> (0, 0) construction
  arc A11 (-5.8792, -32.9801) -> (5.8792, -32.9801) centre (0, -34.0281) ccw
  line L5 (0, -39) -> (0, -40) construction
  arc A12 (-25.622, 21.5816) -> (-31.5012, 11.3985) centre (-29.4692, 17.0141) ccw
  line L6 (-25.622, 21.5816) -> (-24.0923, 20.2931) construction
  line L7 (-31.5012, 11.3985) -> (-29.6205, 10.718) construction
  arc A13 (31.5012, 11.3985) -> (25.622, 21.5816) centre (29.4692, 17.0141) ccw
  circle A14 centre (0, 0) radius 34.0281 construction
  circle A15 centre (0, 0) radius 10.75
  dimension "d101" = 5
  dimension "d12" = 67
  dimension "d13" = 4
  dimension "d14" = 30.5
  dimension "d19" = 2
  dimension "d35" = 3
  dimension "d36" = 3
  dimension "d181" = 1
  dimension "d182" = 120
  dimension "d191" = 21.5
  constraints: 22 point on circle, 15 centre point, 14 end point, 10 coincident, 6 point on line, 5 equal radius, 4 tangent, 1 vertical alignment, 4 other
  measures "d12" diameter of A1
  measures "d13" diameter of A0
  measures "d14" diameter of A2
  measures "d19" radial gap between concentric circles of A1 A3
  measures "d35" diameter of A4
  measures "d36" radial gap between concentric circles of A7 A1
  measures "d181" distance of L5.end L5.start
  measures "d182" angle of L4 L3
  measures "d191" diameter of A15
extrude "Extrusion1" add sketch "Enclosure" along normal blind 4 contours A1 | A3
extrude "Extrusion2" cut sketch "Riemen" along normal blind 3
ref_plane "Arbeitsebene1" through (0, 0, -34) normal (0, 0, 1) x (1, 0, 0)
extrude "Extrusion7" add sketch "Enclosure" along normal blind 2 from surface at -34 contours A1 A13 | A11 A1 | A1 A12 | A8 | A9 | A10
sketch "Skizze4" plane through (0, 0, -34) normal (0, 0, -1) x (-1, 0, 0)
  circle A0 centre (0, 0) radius 10.5
  circle A1 centre (0, 0) radius 9.5
  circle A2 centre (0, 0) radius 5
  circle A3 centre (0, 0) radius 33.5 projected
  circle A4 centre (0, 0) radius 33.5 projected
  circle A5 centre (0, 0) radius 33.5 projected
  circle A6 centre (0, 0) radius 33.5 projected
  circle A7 centre (0, 0) radius 33.5 projected
  arc A8 (-33.5, 0) -> (-33.5, 0) centre (-32.1073, 5.7113) ccw
  circle A9 centre (-31.6099, 18.25) radius 1.5 projected
  circle A10 centre (0, -36.5) radius 1.5 projected
  circle A11 centre (31.6099, 18.25) radius 1.5 projected
  line L0 (0, -54.7) -> (0, 48.2) construction
  line L1 (-52.6777, 0) -> (52.6777, 0) construction
  arc A12 (-33.5, 0) -> (-33.5, 0) centre (-32.1073, 5.7113) ccw
  arc A13 (31.5012, 11.3985) -> (25.622, 21.5816) centre (29.4692, 17.0141) ccw projected
  arc A14 (-25.622, 21.5816) -> (-31.5012, 11.3985) centre (-29.4692, 17.0141) ccw projected
  arc A15 (-5.8792, -32.9801) -> (5.8792, -32.9801) centre (0, -34.0281) ccw projected
  circle A16 centre (0, -36.5) radius 2.5 projected
  circle A17 centre (-31.6099, 18.25) radius 2.5 projected
  circle A18 centre (31.6099, 18.25) radius 2.5 projected
  circle A19 centre (0, 0) radius 33.5 projected
  circle A20 centre (0, 0) radius 31.5 projected
  line L2 (29.2902, -18.23) -> (28.4413, -17.7016) construction
  point P0 (0, 33.5)
  dimension "d22" = 21
  dimension "d23" = 19
  dimension "d45" = 10
  dimension "d241" = 1
  constraints: 5 centre point, 4 point on circle, 3 coincident, 2 end point, 1 point on line, 4 other
  measures "d22" diameter of A0
  measures "d23" diameter of A1
  measures "d45" diameter of A2
  measures "d241" distance of L2.start L2.end
extrude "Extrusion4" add sketch "Skizze4" along normal blind 2 separate body contours A3 A8 A20 | A3 A13 | A15 A3 | A3 A8 A14 | A3 A8 A20 | A3 A14 A8 | A20 A8 | A8 A20 | A16 | A17 | A18 picked at (-28.0603, 20.0861) picked at (-31.5858, 11.4923)
extrude "Extrusion5" add sketch "Skizze4" along normal blind 5 contours A0 bodies 2
extrude "Extrusion6" add sketch "Skizze4" against normal blind 4 from surface at 5 contours A0 | A1 bodies 2
extrude "Extrusion8" add sketch "Enclosure" against normal up to surface (34 mm away) contours A1 bodies 1
ref_plane "Arbeitsebene10" through (0, 0, -16) normal (0, 0, 1) x (1, 0, 0)
sketch "Holes" plane through (0, 0, -16) normal (0, 0, 1) x (1, 0, 0)
  line L0 (0, 250.5339) -> (0, -318.2557) construction
  line L1 (-57.6228, 0) -> (60.6692, 0) construction
  line L2 (-22.5, 35.1536) -> (22.5, 35.1536)
  line L3 (-19.1939, -37.0624) -> (-41.6939, 1.9088)
  line L4 (41.6939, 1.9088) -> (19.1939, -37.0624)
  line L5 (-22.5, 12.9904) -> (-22.5, 35.1536)
  line L6 (22.5, 35.1536) -> (22.5, 12.9904)
  circle A0 centre (0, 0) radius 33.5 construction
  line L7 (-41.6939, 1.9088) -> (-22.5, 12.9904)
  line L8 (-19.1939, -37.0624) -> (0, -25.9808)
  line L9 (19.1939, -37.0624) -> (0, -25.9808)
  line L10 (41.6939, 1.9088) -> (22.5, 12.9904)
  line L11 (0, -25.9808) -> (22.5, 12.9904) construction
  line L12 (0, -25.9808) -> (-22.5, 12.9904) construction
  line L13 (0, 0) -> (22.5, 12.9904) construction
  line L14 (-11.25, -6.4952) -> (0, 0) construction
  circle A1 centre (0, 0) radius 25.9808
  dimension "d123" = 45
  constraints: 26 end point, 6 perpendicular, 4 equal length, 3 point on circle, 1 centre point, 1 coincident, 1 collinear, 1 midpoint, 1 parallel, 1 point on line, 1 other
  measures "d123" distance of L2.start L2.end
extrude "Extrusion33" cut sketch "Holes" along normal mid plane 25 contours L2 L6 A1 L5 | A1 L8 L3 L7 | L10 L4 L9 A1 bodies 1
ref_plane "Arbeitsebene13" through (0, 0, -25) normal (0, 0, -1) x (-1, 0, 0)